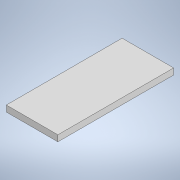
# Autodesk Inventor part: piastra_motore
Saved by Autodesk Inventor 2022 (Build 260153000, 153)
## iProperties
Created: 2022-08-22
Part Number: piastra_motore
Material: Generico
Document SubType Name: Modeling
Designer: matte
Density: 1 g/cm^3
Appearance: Default
Author: matte
Autodesk Inventor part; units mm, degrees
ref_plane "YZ Plane" through (0, 0, 0) normal (1, 0, 0) x (0, 1, 0)
ref_plane "XZ Plane" through (0, 0, 0) normal (0, 1, 0) x (-1, 0, 0)
ref_plane "XY Plane" through (0, 0, 0) normal (0, 0, 1) x (1, 0, 0)
sketch "Schizzo1" plane through (0, 0, 0) normal (0, 1, 0) x (-1, 0, 0)
  line L0 (12.2119, 23.2568) -> (-4.6185, 23.2568)
  line L1 (-4.6185, 23.2568) -> (-4.6185, -14.5458)
  line L2 (-4.6185, -14.5458) -> (12.2119, -14.5458)
  line L3 (12.2119, -14.5458) -> (12.2119, 23.2568)
  point P0 (0, 0)
  constraints: 8 end point, 2 parallel, 1 horizontal, 1 perpendicular
extrude "Estrusione1" add sketch "Schizzo1" along normal blind 2
